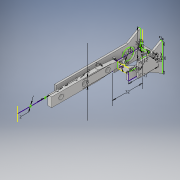
# Autodesk Inventor part: sampleholder6
Saved by Autodesk Inventor 2019 (Build 230136000, 136)
## iProperties
Created: 2019-02-19
Part Number: sampleholder6
Material: Generic
Document SubType Name: Modeling
Designer: rhaase
Density: 1 g/cm^3
Appearance: Default
Author: rhaase
Autodesk Inventor part; units mm, degrees
ref_plane "YZ Plane" through (0, 0, 0) normal (1, 0, 0) x (0, 1, 0)
ref_plane "XZ Plane" through (0, 0, 0) normal (0, 1, 0) x (-1, 0, 0)
ref_plane "XY Plane" through (0, 0, 0) normal (0, 0, 1) x (1, 0, 0)
sketch "Sketch1" plane through (0, 0, 0) normal (0, 0, 1) x (1, 0, 0)
  line L0 (0, 0) -> (8.5, 0)
  line L1 (8.5, 0) -> (8.5, 1)
  line L2 (8.5, 1) -> (-8.5, 1)
  line L3 (-8.5, 1) -> (-8.5, -1)
  line L4 (-8.5, -1) -> (8.5, -1)
  line L5 (8.5, -1) -> (8.5, 1)
  circle A0 centre (0, 0) radius 1
  line L6 (-8.5, 0) -> (-7.5, 0)
  line L7 (8.5, 0) -> (7.5, 0)
  circle A1 centre (-7.5, 0) radius 1
  circle A2 centre (7.5, 0) radius 1
  line L8 (-7.5, 0) -> (-7.5, 2)
  line L9 (-7.5, 0) -> (-7.5, -2)
  line L10 (7.5, 0) -> (7.5, 2)
  line L11 (7.5, 0) -> (7.5, -2)
  line L12 (8.5, 2) -> (6.5, 2)
  line L13 (6.5, 2) -> (6.5, -2)
  line L14 (6.5, -2) -> (8.5, -2)
  line L15 (8.5, -2) -> (8.5, 2)
  line L16 (-8.5, 2) -> (-6.5, 2)
  line L17 (-6.5, 2) -> (-6.5, -2)
  line L18 (-6.5, -2) -> (-8.5, -2)
  line L19 (-8.5, -2) -> (-8.5, 2)
  circle A3 centre (-7.5, 2) radius 1
  circle A4 centre (-7.5, -2) radius 1
  circle A5 centre (7.5, -2) radius 1
  circle A6 centre (7.5, 2) radius 1
  dimension "d3" = 8.5
  dimension "d4" = 1
  dimension "d5" = 17
  dimension "d6" = 2
  dimension "d7" = 2
  dimension "d8" = 1
  dimension "d9" = 1
  dimension "d10" = 2
  dimension "d11" = 2
  dimension "d12" = 2
  dimension "d13" = 2
  dimension "d14" = 2
  dimension "d15" = 2
  dimension "d16" = 2
  dimension "d17" = 2
  constraints: 40 end point, 7 coincident, 6 parallel, 5 centre point, 5 horizontal, 5 perpendicular, 3 point on line, 3 vertical, 2 horizontal alignment, 1 midpoint, 4 other
  measures "d3" distance of L0.start L0.end
  measures "d4" distance of L0.end L1.end
  measures "d5" distance of L4.end L3.end
  measures "d6" distance of L3.end L2.end
  measures "d7" diameter of A0
  measures "d8" distance of L6.start L6.end
  measures "d9" distance of L0.end L7.end
  measures "d10" distance of L8.start L8.end
  measures "d11" distance of L8.start L9.end
  measures "d12" distance of L10.start L10.end
  measures "d13" distance of L10.start L11.end
  measures "d14" diameter of A3
  measures "d15" diameter of A4
  measures "d16" diameter of A5
  measures "d17" diameter of A6
extrude "Extrusion1" add sketch "Sketch1" along normal blind 25 contours A6 L12 L10 | L10 L12 A6 | A5 L14 L11 | L11 L14 A5 | L12 A6 | L14 A5 | A3 L16 L8 | L8 L16 A3 | L16 A3 | A4 L18 L9 | L9 L18 A4 | A4 L18
extrude "Extrusion2" add sketch "Sketch1" against normal blind 3
extrude "Extrusion3" add sketch "Sketch1" along normal blind 6 contours A0
sketch "Sketch2" plane through (0, 0, 6) normal (0, 0, 1) x (1, 0, 0)
  circle A0 centre (0, 0) radius 0.65
  dimension "d25" = 1.3
  constraints: 1 centre point
  measures "d25" diameter of A0
extrude "Extrusion4" cut sketch "Sketch2" against normal blind 2
sketch "Sketch3" plane through (7.5, 2, 25) normal (0, 0, 1) x (1, 0, 0)
  circle A0 centre (0, 0) radius 1 projected
  arc A1 (-16, -4) -> (-14, -4) centre (-15, -4) ccw projected
  line L0 (0, 1) -> (-15, 1)
  line L1 (-15, 1) -> (-15, -5)
  line L2 (-15, -5) -> (0, -5)
  line L3 (0, -5) -> (0, 1)
  line L4 (1, -4) -> (1, 0) projected
  arc A2 (-16, 0) -> (-14, 0) centre (-15, 0) ccw projected
  line L5 (1, -4) -> (-16, -4)
  line L6 (-16, -4) -> (-16, 0)
  line L7 (-16, 0) -> (1, 0)
  line L8 (1, 0) -> (1, -4)
  circle A3 centre (0, -4) radius 1 projected
  circle A4 centre (0, -4) radius 1
  circle A5 centre (0, 0) radius 1
  circle A6 centre (-15, 0) radius 1 projected
  circle A7 centre (-15, 0) radius 1
  circle A8 centre (-15, -4) radius 1
  point P0 (-7.5, -2)
  constraints: 16 end point, 4 coincident, 4 parallel, 2 centre point, 2 horizontal, 2 perpendicular, 2 point on circle, 2 vertical alignment, 4 other
sketch "Sketch4" plane through (-7.5, 2, 25) normal (0, 0, 1) x (1, 0, 0)
  point P0 (7.5, -2)
extrude "Extrusion5" add sketch "Sketch3" along normal blind 3
sketch "Sketch5" plane through (-7.5, -3, 25) normal (0, -1, 0) x (1, 0, 0)
  line L0 (15, 0) -> (15, 3) projected
  line L1 (15, 3) -> (15, -9)
  line L2 (15, -9) -> (6, 0)
  line L3 (15, 0) -> (0, 0) projected
  line L4 (6, 0) -> (15, 3)
  line L5 (0, 3) -> (0, -9)
  line L6 (0, -9) -> (9, 0)
  line L7 (15, 3) -> (0, 3) projected
  line L8 (9, 0) -> (0, 3)
  point P0 (7.5, -25)
  dimension "d30" = 12
  dimension "d31" = 45
  dimension "d32" = 45
  constraints: 12 end point, 2 point on line, 1 collinear, 1 vertical
  measures "d30" distance of L0.end L1.end
  measures "d31" angle of L1 L2
  measures "d32" angle of L6 L5
extrude "Extrusion6" add sketch "Sketch5" against normal blind 2 contours L1 L2 L6 L3 | L6 L2 L3 | L3 L4 L8 | L4 L3 L5 L8 | L6 L5 L3 L2
sketch "Sketch6" plane through (-7.5, 3, 25) normal (0, 1, 0) x (1, 0, 0)
  line L0 (-1, -3) -> (0, -3) projected
  line L1 (0, -3) -> (0, 9)
  line L2 (-1, 28) -> (-1, -3) projected
  line L3 (0, -3) -> (12, -3) construction
  line L4 (0, 9) -> (9, 0)
  line L5 (15, 0) -> (0, 0) projected
  line L6 (0, -3) -> (15, -3) projected
  line L7 (9, 0) -> (0, -3)
  line L8 (15, 9) -> (15, 0) projected
  line L9 (15, -3) -> (15, 9)
  line L10 (15, 9) -> (3, -3)
  point P0 (7.5, 25)
  dimension "d35" = 12
  dimension "d36" = 90
  dimension "d37" = 45
  constraints: 12 end point, 2 point on line, 1 collinear, 1 horizontal, 1 parallel, 1 perpendicular
  measures "d35" distance of L0.end L1.end
  measures "d36" angle of L3 L1
  measures "d37" angle of L1 L4
extrude "Extrusion7" add sketch "Sketch6" against normal blind 2 contours L1 L4 L10 L5 | L10 L7 L5 L9 L6 | L10 L5 L7 | L10 L4 L5 | L4 L10 L8 L5
sketch "Sketch7" plane through (7.5, 2, 28) normal (0, 0, 1) x (1, 0, 0)
  circle A0 centre (-7.5, -2) radius 0.65 projected
  circle A1 centre (-7.5, -2) radius 0.9
  line L0 (0, 1) -> (-15, 1) projected
  line L1 (-16, -5) -> (-12, -5)
  line L2 (-12, -5) -> (-12, 1)
  line L3 (-12, 1) -> (-16, 1)
  line L4 (-16, 1) -> (-16, -5)
  dimension "d40" = 1.8
  dimension "d41" = 4
  constraints: 8 end point, 2 parallel, 1 centre point, 1 coincident, 1 horizontal, 1 perpendicular, 1 point on line
  measures "d40" diameter of A1
  measures "d41" distance of L3.end L2.end
extrude "Extrusion8" cut sketch "Sketch7" against normal blind 10 contours A0 | A1
extrude "Extrusion9" add sketch "Sketch7" along normal blind 60 contours L2 L1 L4 L3 L0
sketch "Sketch10" plane through (0, 0, -3) normal (0, 0, -1) x (-1, 0, 0)
  line L0 (8.5, -3.0252) -> (10.5, -3.0252)
  line L1 (10.5, -3.0252) -> (10.5, 2.9748)
  line L2 (10.5, 2.9748) -> (8.5, 2.9748)
  line L3 (8.5, 2.9748) -> (8.5, -3.0252)
  line L4 (-8.5, 3) -> (-10.5, 3)
  line L5 (-10.5, 3) -> (-10.5, -3)
  line L6 (-10.5, -3) -> (-8.5, -3)
  line L7 (-8.5, -3) -> (-8.5, 3)
  line L8 (10.5, 15) -> (12.5, 15)
  line L9 (12.5, 15) -> (12.5, -15)
  line L10 (12.5, -15) -> (10.5, -15)
  line L11 (10.5, -15) -> (10.5, 15)
  line L12 (-10.5, -15) -> (-12.5, -15)
  line L13 (-12.5, -15) -> (-12.5, 15)
  line L14 (-12.5, 15) -> (-10.5, 15)
  line L15 (-10.5, 15) -> (-10.5, -15)
  point P0 (0, 0)
  dimension "d62" = 2
  dimension "d63" = 6
  dimension "d64" = 2
  dimension "d65" = 6
  dimension "d66" = 2
  dimension "d67" = 30
  dimension "d68" = 2
  dimension "d69" = 30
  constraints: 32 end point, 8 parallel, 4 horizontal, 4 perpendicular, 3 point on line
  measures "d62" distance of L2.end L1.end
  measures "d63" distance of L1.end L0.end
  measures "d64" distance of L6.end L5.end
  measures "d65" distance of L5.end L4.end
  measures "d66" distance of L9.end L10.end
  measures "d67" distance of L8.end L9.end
  measures "d68" distance of L13.end L14.end
  measures "d69" distance of L12.end L13.end
extrude "Extrusion12" add sketch "Sketch10" against normal blind 25 contours L5 L15 L12 L13 L14
extrude "Extrusion13" add sketch "Sketch10" against normal blind 130 contours L1 L11 L8 L9 L10
sketch "Sketch11" plane through (-12.5, -15, -3) normal (-1, 0, 0) x (0, 0, 1)
  point P0 (3, 15)
sketch "Sketch12" plane through (-12.5, -15, -3) normal (-1, 0, 0) x (0, 0, 1)
  line L0 (0, 30) -> (0, 0) projected
  line L1 (0, 30) -> (13.3686, 22.2816)
  line L2 (0, 30) -> (15.4368, 30) construction
  line L3 (0, 0) -> (130, 0) projected
  line L4 (0, 0) -> (13.3686, 7.7184)
  line L5 (0, 0) -> (15.4368, 0) construction
  line L6 (13.3686, 7.7184) -> (13.3686, 22.2816)
  line L7 (13.3686, 22.2816) -> (130, 22.2816)
  line L8 (130, 30) -> (130, 0) projected
  line L9 (130, 7.7184) -> (13.3686, 7.7184)
  line L10 (0, 0) -> (130, 0)
  line L11 (130, 7.7184) -> (130, 22.2816)
  line L12 (130, 30) -> (0, 30)
  point P0 (3, 15)
  dimension "d74" = 30
  dimension "d75" = 30
  constraints: 20 end point, 4 horizontal, 2 equal length, 2 perpendicular, 1 collinear, 1 parallel, 1 point on line
  measures "d74" angle of L1 L2
  measures "d75" angle of L5 L4
extrude "Extrusion14" cut sketch "Sketch12" against normal blind 130 contours L12 L8 L7 L1 | L4 L9 L8 L3
sketch "Sketch13" plane through (-12.5, -15, -3) normal (-1, 0, 0) x (0, 0, 1)
  line L0 (0, 30) -> (0, 0) projected
  line L1 (0, 15) -> (130, 15)
  line L2 (130, 22.2816) -> (130, 7.7184) projected
  circle A0 centre (40, 15) radius 1
  circle A1 centre (60, 15) radius 1
  circle A2 centre (80, 15) radius 1
  circle A3 centre (100, 15) radius 1
  circle A4 centre (115.7268, 15) radius 1
  point P0 (3, 15)
  dimension "d79" = 2
  dimension "d80" = 2
  dimension "d81" = 2
  dimension "d82" = 2
  dimension "d83" = 2
  constraints: 5 centre point, 4 point on line, 2 end point, 2 midpoint
  measures "d79" diameter of A0
  measures "d80" diameter of A1
  measures "d81" diameter of A2
  measures "d82" diameter of A3
  measures "d83" diameter of A4
sketch "Sketch18" plane through (-4.5, -3, 28) normal (1, 0, 0) x (0, 0, -1)
  line L0 (-20, 8.0747) -> (-70, 8.0747)
  line L1 (-70, 8.0747) -> (-70, -1.9253)
  line L2 (-70, -1.9253) -> (-20, -1.9253)
  line L3 (-20, -1.9253) -> (-20, 8.0747)
  point P0 (28, 3)
  dimension "d106" = 50
  dimension "d107" = 10
  constraints: 8 end point, 2 parallel, 1 horizontal, 1 perpendicular
  measures "d106" distance of L2.end L1.end
  measures "d107" distance of L1.end L0.end
extrude "Extrusion21" add sketch "Sketch18" against normal blind 4
sketch "Sketch19" plane through (-4.5, -3, 28) normal (1, 0, 0) x (0, 0, -1)
  line L0 (-70, 8.0747) -> (-20, 8.0747) projected
  line L1 (0, 6) -> (-20, 8.0747)
  line L2 (-20, 6) -> (-20, 8.0747) projected
  line L3 (-20, 8.0747) -> (-20, 6)
  line L4 (0, 6) -> (-20, 6) projected
  line L5 (-20, 6) -> (0, 6)
  line L6 (0, 0) -> (-20, 0) projected
  line L7 (-20, -1.9253) -> (-20, 0) projected
  line L8 (0, 0) -> (-20, -1.9253)
  line L9 (-20, -1.9253) -> (-20, 0)
  line L10 (0, 1) -> (0, 0) projected
  line L11 (-20, 0) -> (0, 0)
  point P0 (28, 3)
  constraints: 12 end point, 2 perpendicular
extrude "Extrusion22" add sketch "Sketch19" against normal blind 4
sketch "Sketch20" plane through (-4.5, -4.9253, 98) normal (1, 0, 0) x (0, 0, -1)
  circle A0 centre (60, 5) radius 2.5
  line L0 (60, 5) -> (35, 5)
  circle A1 centre (35, 5) radius 2.5
  line L1 (35, 5) -> (10, 5)
  circle A2 centre (10, 5) radius 2.5
  point P0 (98, 4.9253)
  dimension "d112" = 5
  dimension "d113" = 25
  dimension "d114" = 5
  dimension "d115" = 25
  dimension "d116" = 5
  constraints: 4 end point, 3 centre point, 2 coincident, 2 horizontal
  measures "d112" diameter of A0
  measures "d113" distance of L0.start L0.end
  measures "d114" diameter of A1
  measures "d115" distance of L1.start L1.end
  measures "d116" diameter of A2
extrude "Extrusion23" cut sketch "Sketch20" against normal blind 4
sketch "Sketch21" plane through (7.5, 3, 28) normal (0, 1, 0) x (1, 0, 0)
  line L0 (1, 31) -> (1, 0) projected
  line L1 (1, 22.4049) -> (3, 22.4049)
  line L2 (3, 22.4049) -> (3, 20.4049)
  line L3 (3, 20.4049) -> (1, 20.4049)
  line L4 (1, 20.4049) -> (1, 22.4049)
  line L5 (-16.0375, 20.4049) -> (-18.0375, 20.4049)
  line L6 (-18.0375, 20.4049) -> (-18.0375, 22.4049)
  line L7 (-18.0375, 22.4049) -> (-16.0375, 22.4049)
  line L8 (-16.0375, 22.4049) -> (-16.0375, 20.4049)
  line L9 (-16, 31) -> (-16, 0) projected
  line L10 (-16, 11.5515) -> (-18, 11.5515)
  line L11 (-18, 11.5515) -> (-18, 13.5515)
  line L12 (-18, 13.5515) -> (-16, 13.5515)
  line L13 (-16, 13.5515) -> (-16, 11.5515)
  line L14 (1, 11.5515) -> (3, 11.5515)
  line L15 (3, 11.5515) -> (3, 13.5515)
  line L16 (3, 13.5515) -> (1, 13.5515)
  line L17 (1, 13.5515) -> (1, 11.5515)
  line L18 (3, 6) -> (3, 17.6314) projected
  line L19 (3, 6) -> (1, 6)
  line L20 (1, 6) -> (1, 8)
  line L21 (1, 8) -> (3, 8)
  line L22 (3, 8) -> (3, 6)
  line L23 (-16, 0.6981) -> (-18, 0.6981)
  line L24 (-18, 0.6981) -> (-18, 2.6981)
  line L25 (-18, 2.6981) -> (-16, 2.6981)
  line L26 (-16, 2.6981) -> (-16, 0.6981)
  line L27 (-16, -20) -> (-16, 0) projected
  line L28 (-16, -20) -> (-18, -20)
  line L29 (-18, -20) -> (-18, -22)
  line L30 (-18, -22) -> (-16, -22)
  line L31 (-16, -22) -> (-16, -20)
  line L32 (-18, 17.6314) -> (-18, -99) projected
  line L33 (-18, -40.6843) -> (-16, -40.6843)
  line L34 (-16, -40.6843) -> (-16, -42.6843)
  line L35 (-16, -42.6843) -> (-18, -42.6843)
  line L36 (-18, -42.6843) -> (-18, -40.6843)
  line L37 (-16, -70) -> (-16, -20) projected
  line L38 (-16, -64.5869) -> (-18, -64.5869)
  line L39 (-18, -64.5869) -> (-18, -66.0669)
  line L40 (-18, -66.0669) -> (-16, -66.0669)
  line L41 (-16, -66.0669) -> (-16, -64.5869)
  dimension "d131" = 2
  dimension "d132" = 2
  dimension "d133" = 2
  dimension "d134" = 2
  dimension "d135" = 2
  dimension "d136" = 2
  dimension "d137" = 2
  dimension "d138" = 2
  dimension "d139" = 2
  dimension "d140" = 2
  dimension "d141" = 2
  dimension "d142" = 2
  dimension "d143" = 2
  dimension "d144" = 2
  dimension "d145" = 2
  dimension "d146" = 2
  constraints: 72 end point, 18 parallel, 9 horizontal, 9 perpendicular, 8 point on line, 2 other
  measures "d131" distance of L2.end L3.end
  measures "d132" distance of L1.end L2.end
  measures "d133" distance of L6.end L7.end
  measures "d134" distance of L5.end L6.end
  measures "d135" distance of L11.end L12.end
  measures "d136" distance of L10.end L11.end
  measures "d137" distance of L16.end L15.end
  measures "d138" distance of L15.end L14.end
  measures "d139" distance of L20.end L21.end
  measures "d140" distance of L19.end L20.end
  measures "d141" distance of L24.end L25.end
  measures "d142" distance of L23.end L24.end
  measures "d143" distance of L30.end L29.end
  measures "d144" distance of L29.end L28.end
  measures "d145" distance of L34.end L35.end
  measures "d146" distance of L33.end L34.end
extrude "Extrusion24" add sketch "Sketch21" against normal blind 2 contours L1 L2 L3 L0 | L16 L15 L14 L0 | L21 L18 L19 L0 | L5 L6 L7 L8 | L9 L10 L11 L12 | L9 L23 L24 L25 | L31 L30 L29 L28 | L34 L35 L32 L33 | L37 L40 L32 L38
sketch "Sketch22" plane through (7.5, -3, 16) normal (0, -1, 0) x (1, 0, 0)
  line L0 (-18, -10.4049) -> (-16.0375, -10.4049) projected
  line L1 (-18, -10.4049) -> (-16, -10.4049)
  line L2 (-16, -10.4049) -> (-16, -8.4049)
  line L3 (-16, -8.4049) -> (-18, -8.4049)
  line L4 (-18, -8.4049) -> (-18, -10.4049)
  line L5 (3, -5.6314) -> (3, -19) projected
  line L6 (3, -10.4049) -> (1, -10.4049)
  line L7 (1, -10.4049) -> (1, -8.4049)
  line L8 (1, -8.4049) -> (3, -8.4049)
  line L9 (3, -8.4049) -> (3, -10.4049)
  line L10 (3, 6) -> (3, -5.6314) projected
  line L11 (3, -1.5292) -> (1, -1.5292)
  line L12 (1, -1.5292) -> (1, 0.4708)
  line L13 (1, 0.4708) -> (3, 0.4708)
  line L14 (3, 0.4708) -> (3, -1.5292)
  line L15 (-18, 0.4708) -> (-16, 0.4708)
  line L16 (-16, 0.4708) -> (-16, -1.5292)
  line L17 (-16, -1.5292) -> (-18, -1.5292)
  line L18 (-18, -1.5292) -> (-18, 0.4708)
  point P0 (-7.5, -16)
  dimension "d149" = 2
  dimension "d150" = 2
  dimension "d151" = 2
  dimension "d152" = 2
  dimension "d153" = 2
  dimension "d154" = 2
  dimension "d155" = 2
  dimension "d156" = 2
  constraints: 32 end point, 8 parallel, 5 point on line, 4 horizontal, 4 perpendicular
  measures "d149" distance of L3.end L2.end
  measures "d150" distance of L2.end L1.end
  measures "d151" distance of L7.end L8.end
  measures "d152" distance of L6.end L7.end
  measures "d153" distance of L12.end L13.end
  measures "d154" distance of L11.end L12.end
  measures "d155" distance of L16.end L17.end
  measures "d156" distance of L15.end L16.end
extrude "Extrusion25" add sketch "Sketch22" against normal blind 2
sketch "Sketch23" plane through (-10.5, -15, -3) normal (1, 0, 0) x (0, 0, -1)
  line L0 (-130, 7.7184) -> (-130, 22.2816) projected
  line L1 (-130, 7.7184) -> (-90, 7.7184)
  line L2 (-90, 7.7184) -> (-90, 22.7184)
  line L3 (-90, 22.7184) -> (-130, 22.7184)
  line L4 (-130, 22.7184) -> (-130, 7.7184)
  point P0 (-3, 15)
  dimension "d159" = 40
  dimension "d160" = 15
  constraints: 8 end point, 2 parallel, 1 horizontal, 1 perpendicular
  measures "d159" distance of L3.end L2.end
  measures "d160" distance of L2.end L1.end
extrude "Extrusion26" cut sketch "Sketch23" against normal blind 5
sketch "Sketch24" plane through (-8.5, -3, 16.4708) normal (1, 0, 0) x (0, 0, -1)
  point P0 (16.4708, 3)
sketch "Sketch25" plane through (-8.5, -3, 7.5951) normal (1, 0, 0) x (0, 0, -1)
  line L0 (10.5951, 18) -> (10.5951, -12) projected
  line L1 (10.5951, 3) -> (-21.4049, 3)
  line L2 (-21.4049, 3) -> (-21.4049, -5)
  line L3 (-21.4049, -5) -> (10.5951, -5)
  line L4 (10.5951, -5) -> (10.5951, 3)
  circle A0 centre (-5, 3) radius 6
  point P0 (7.5951, 3)
  dimension "d163" = 32
  dimension "d164" = 8
  dimension "d165" = 12
  constraints: 8 end point, 2 parallel, 1 centre point, 1 horizontal, 1 midpoint, 1 perpendicular
  measures "d163" distance of L3.end L2.end
  measures "d164" distance of L2.end L1.end
  measures "d165" diameter of A0
extrude "Extrusion27" add sketch "Sketch25" along normal blind 2 contours L0 L3 L2 L1 A0 | A0 L1 picked at (-6.668, 0.2657)
extrude "Extrusion28" cut sketch "Sketch25" along normal blind 2 contours A0 L1 | L1 A0
sketch "Sketch26" plane through (8.5, -3, 5.5951) normal (-1, 0, 0) x (0, 0, 1)
  line L0 (-8.5951, -5) -> (-8.5951, 5) projected
  line L1 (23.4049, -0.0963) -> (23.4049, -5) projected
  line L2 (-8.5951, 3) -> (23.4049, 3)
  line L3 (23.4049, 3) -> (23.4049, -5)
  line L4 (23.4049, -5) -> (-8.5951, -5)
  line L5 (-8.5951, -5) -> (-8.5951, 3)
  circle A0 centre (7, 3) radius 6
  point P0 (-5.5951, 3)
  dimension "d170" = 32
  dimension "d171" = 12
  constraints: 8 end point, 2 parallel, 2 point on line, 1 centre point, 1 horizontal, 1 perpendicular
  measures "d170" distance of L1.end L4.end
  measures "d171" diameter of A0
extrude "Extrusion29" add sketch "Sketch26" along normal blind 2 contours L0 L2 A0 L3 L1 L4 | L2 A0 picked at (5.8639, 1.354)
extrude "Extrusion30" cut sketch "Sketch26" along normal blind 2 contours A0 L2 | L2 A0
sketch "Sketch27" plane through (8.5, 2, 0) normal (1, 0, 0) x (0, 0, -1)
  line L0 (-28, -2) -> (-28, 0) projected
  line L1 (-28, -2) -> (-12, -2)
  line L2 (-12, -2) -> (-12, 1)
  line L3 (-12, 1) -> (-28, 1)
  line L4 (-28, 1) -> (-28, -2)
  line L5 (-18.5951, -2) -> (-25, -2) projected
  line L6 (-28, 1) -> (-25, -2)
  line L7 (-25, -2) -> (-12, -2)
  point P0 (0, -2)
  dimension "d176" = 16
  constraints: 12 end point, 2 parallel, 1 collinear, 1 horizontal, 1 perpendicular
  measures "d176" distance of L3.end L2.end
extrude "Extrusion31" cut sketch "Sketch27" against normal blind 17 contours L6 L3 L2 L1
sketch "Sketch28" plane through (0, 0, -3) normal (0, 0, -1) x (-1, 0, 0)
  line L0 (-8.5, 0) -> (-8.5, 2) projected
  line L1 (7.5, 3) -> (8.5, 3) projected
  line L2 (-8.5, 1) -> (8.5, 1)
  line L3 (8.5, 1) -> (8.5, 3)
  line L4 (8.5, 3) -> (-8.5, 3)
  line L5 (-8.5, 3) -> (-8.5, 1)
  point P0 (0, 0)
  constraints: 8 end point, 2 parallel, 1 horizontal, 1 midpoint, 1 perpendicular
extrude "Extrusion32" cut sketch "Sketch28" against normal blind 17
sketch "Sketch29" plane through (10.5, -15, -3) normal (-1, 0, 0) x (0, 0, 1)
  line L0 (25, 16) -> (25, 7.7184) projected
  line L1 (25, 13.7944) -> (26, 13.7944)
  line L2 (26, 13.7944) -> (26, 14.7944)
  line L3 (26, 14.7944) -> (25, 14.7944)
  line L4 (25, 14.7944) -> (25, 13.7944)
  point P0 (3, 15)
  dimension "d181" = 1
  dimension "d182" = 1
  constraints: 8 end point, 2 parallel, 1 horizontal, 1 perpendicular, 1 point on line
  measures "d181" distance of L3.end L2.end
  measures "d182" distance of L2.end L1.end
extrude "Extrusion33" add sketch "Sketch29" along normal mid plane 4
body "Solid1"
